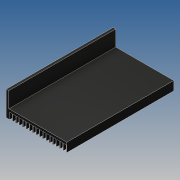
# Autodesk Inventor part: 800-20-MOTOR-CONTROLLER-BLD-300B-01
Saved by Autodesk Inventor 2018.2 (Build 222227000, 227)
## iProperties
Manager: feesmrt
Company: FRANCOR
Part Number: 800-20-MOTOR-CONTROLLER-BLD-300B-01
Material: Aluminium 6061
Document SubType Name: Modeling
Designer: feesmrt
Density: 2.7 g/cm^3
Appearance: Glänzend - schwarz
Project: Rescue Robot
Cost Center: -
Engineer: feesmrt
Authority: feesmrt
Description: BLDC Motor Driver BLD-300B - Kühler
Stock Number: 800-20-MOTOR-CONTROLLER-BLD-300B-01
Author: feesmrt
Subject: Rescue Robot
Revision Number: 1
Title: BLDC Motor Driver BLD-300B - Kühler
Autodesk Inventor part; units mm, degrees
ref_plane "YZ Plane" through (0, 0, 0) normal (1, 0, 0) x (0, 1, 0)
ref_plane "XZ Plane" through (0, 0, 0) normal (0, 1, 0) x (-1, 0, 0)
ref_plane "XY Plane" through (0, 0, 0) normal (0, 0, 1) x (1, 0, 0)
sketch "Skizze1" plane through (0, 0, 0) normal (0, 0, 1) x (1, 0, 0)
  line L0 (-40.5, -71.5) -> (40.5, -71.5)
  line L1 (40.5, -71.5) -> (40.5, 71.5)
  line L2 (40.5, 71.5) -> (-40.5, 71.5)
  line L3 (-40.5, 71.5) -> (-40.5, -71.5)
  line L4 (-40.5, -71.5) -> (40.5, 71.5) construction
  line L5 (40.5, -71.5) -> (-40.5, 71.5) construction
  point P0 (0, 0)
  dimension "d0" = 143
  dimension "d1" = 81
  constraints: 12 end point, 2 midpoint, 2 parallel, 1 horizontal, 1 perpendicular
  measures "d0" distance of L0.end L1.end
  measures "d1" distance of L1.end L2.end
extrude "Grundkörper" add sketch "Skizze1" along normal blind 33
sketch "Skizze2" plane through (-40.5, -71.5, 0) normal (0, -1, 0) x (1, 0, 0)
  line L0 (0, 0) -> (0, 33) projected
  line L1 (0, 0) -> (81, 0) projected
  line L2 (0, 0) -> (81, 0) projected
  line L3 (81, 0) -> (81, 33) projected
  line L4 (0, 33) -> (81, 33) projected
  line L5 (0, 0) -> (0, 33) projected
  line L6 (81, 0) -> (81, 33) projected
  line L7 (3.5, 33) -> (3.5, 12)
  line L8 (3.5, 12) -> (81, 12)
  point P0 (40.5, 0)
  dimension "d4" = 12
  dimension "d5" = 3.5
  constraints: 4 end point, 2 point on line, 1 perpendicular, 1 vertical
  measures "d4" distance between parallel lines of L1 L8
  measures "d5" distance between parallel lines of L0 L7
extrude "Ausschnitt" cut sketch "Skizze2" against normal through all contours L4 L3 L8 L7
sketch "Skizze3" plane through (-40.5, -71.5, 0) normal (0, -1, 0) x (1, 0, 0)
  line L0 (0, 0) -> (81, 0) construction
  line L1 (81, 0) -> (81, 12) construction
  line L2 (81, 0) -> (0, 0) construction
  line L3 (76.5, 0) -> (80, 0)
  line L4 (80, 0) -> (80, 8.5)
  line L5 (80, 8.5) -> (76.5, 8.5)
  line L6 (76.5, 8.5) -> (76.5, 0)
  line L7 (72, 8.5) -> (72, 0)
  line L8 (72, 0) -> (75.5, 0)
  line L9 (75.5, 0) -> (75.5, 8.5)
  line L10 (75.5, 8.5) -> (72, 8.5)
  line L11 (67.5, 8.5) -> (67.5, 0)
  line L12 (67.5, 0) -> (71, 0)
  line L13 (71, 0) -> (71, 8.5)
  line L14 (71, 8.5) -> (67.5, 8.5)
  line L15 (63, 8.5) -> (63, 0)
  line L16 (63, 0) -> (66.5, 0)
  line L17 (66.5, 0) -> (66.5, 8.5)
  line L18 (66.5, 8.5) -> (63, 8.5)
  line L19 (58.5, 8.5) -> (58.5, 0)
  line L20 (58.5, 0) -> (62, 0)
  line L21 (62, 0) -> (62, 8.5)
  line L22 (62, 8.5) -> (58.5, 8.5)
  line L23 (54, 8.5) -> (54, 0)
  line L24 (54, 0) -> (57.5, 0)
  line L25 (57.5, 0) -> (57.5, 8.5)
  line L26 (57.5, 8.5) -> (54, 8.5)
  line L27 (49.5, 8.5) -> (49.5, 0)
  line L28 (49.5, 0) -> (53, 0)
  line L29 (53, 0) -> (53, 8.5)
  line L30 (53, 8.5) -> (49.5, 8.5)
  line L31 (45, 8.5) -> (45, 0)
  line L32 (45, 0) -> (48.5, 0)
  line L33 (48.5, 0) -> (48.5, 8.5)
  line L34 (48.5, 8.5) -> (45, 8.5)
  line L35 (40.5, 8.5) -> (40.5, 0)
  line L36 (40.5, 0) -> (44, 0)
  line L37 (44, 0) -> (44, 8.5)
  line L38 (44, 8.5) -> (40.5, 8.5)
  line L39 (36, 8.5) -> (36, 0)
  line L40 (36, 0) -> (39.5, 0)
  line L41 (39.5, 0) -> (39.5, 8.5)
  line L42 (39.5, 8.5) -> (36, 8.5)
  line L43 (31.5, 8.5) -> (31.5, 0)
  line L44 (31.5, 0) -> (35, 0)
  line L45 (35, 0) -> (35, 8.5)
  line L46 (35, 8.5) -> (31.5, 8.5)
  line L47 (27, 8.5) -> (27, 0)
  line L48 (27, 0) -> (30.5, 0)
  line L49 (30.5, 0) -> (30.5, 8.5)
  line L50 (30.5, 8.5) -> (27, 8.5)
  line L51 (22.5, 8.5) -> (22.5, 0)
  line L52 (22.5, 0) -> (26, 0)
  line L53 (26, 0) -> (26, 8.5)
  line L54 (26, 8.5) -> (22.5, 8.5)
  line L55 (18, 8.5) -> (18, 0)
  line L56 (18, 0) -> (21.5, 0)
  line L57 (21.5, 0) -> (21.5, 8.5)
  line L58 (21.5, 8.5) -> (18, 8.5)
  line L59 (13.5, 8.5) -> (13.5, 0)
  line L60 (13.5, 0) -> (17, 0)
  line L61 (17, 0) -> (17, 8.5)
  line L62 (17, 8.5) -> (13.5, 8.5)
  line L63 (9, 8.5) -> (9, 0)
  line L64 (9, 0) -> (12.5, 0)
  line L65 (12.5, 0) -> (12.5, 8.5)
  line L66 (12.5, 8.5) -> (9, 8.5)
  line L67 (4.5, 8.5) -> (4.5, 0)
  line L68 (4.5, 0) -> (8, 0)
  line L69 (8, 0) -> (8, 8.5)
  line L70 (8, 8.5) -> (4.5, 8.5)
  point P0 (40.5, 0)
  dimension "d11" = 1
  dimension "d12" = 8.5
  dimension "d13" = 3.5
  dimension "d16" = 4.5
  constraints: 136 end point, 2 horizontal, 2 parallel, 1 perpendicular, 1 point on line, 128 other
  measures "d11" distance between parallel lines of L1 L4
  measures "d12" distance between parallel lines of L0 L5
  measures "d13" distance between parallel lines of L6 L4
  measures "d16" distance of L5.end L7.start
extrude "Kühlrippen" cut sketch "Skizze3" against normal through all
